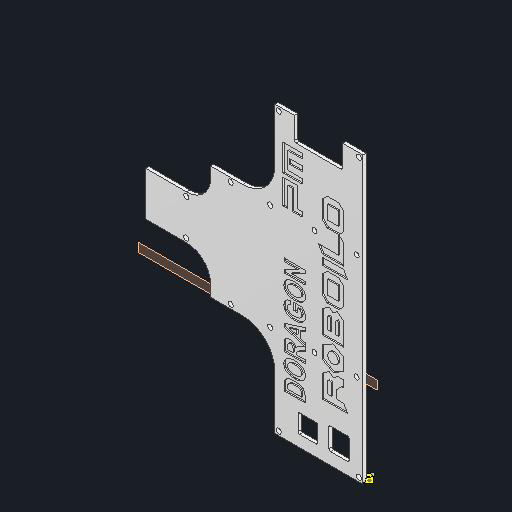
# Autodesk Inventor part: ceil
Saved by Autodesk Inventor 2023 (Build 270158000, 158)
## iProperties
Created: 2024-05-26
Part Number: ceil
Material: ABS Plastic
Document SubType Name: Modeling
Designer: szymo
Density: 1.06 g/cm^3
Appearance: Smooth - White
Mass: 26.6149 g
Surface Area: 293.171 cm^2
Volume: 25.1084 cm^3
TOTAL MASS: 0.0
Author: szymo
Autodesk Inventor part; units mm, degrees
ref_plane "YZ Plane" through (0, 0, 0) normal (1, 0, 0) x (0, 1, 0)
ref_plane "XZ Plane" through (0, 0, 0) normal (0, 1, 0) x (-1, 0, 0)
ref_plane "XY Plane" through (0, 0, 0) normal (0, 0, 1) x (1, 0, 0)
ref_plane "Work Plane1" through (-50.5, 0, 0) normal (0, 0, 1) x (1, 0, 0)
sketch "Sketch3" plane through (-50.5, 0, 0) normal (0, 0, 1) x (1, 0, 0)
  line L0 (135.5648, 0) -> (135.5648, 5.2284) projected
  line L1 (0, 5) -> (134.493, 5) projected
  line L2 (0, 0) -> (0, 5) projected
  line L3 (0, 71) -> (135.5648, 71) projected
  line L4 (0, 71) -> (0, 66) projected
  line L5 (0, 66) -> (135.5648, 66) projected
  line L6 (135.5648, 71) -> (135.5648, 66) projected
  line L7 (131.5648, 119.5) -> (134.5648, 119.5) projected
  line L8 (135.5648, 124.5) -> (135.5648, 120.5) projected
  line L9 (135.5648, 124.5) -> (51.5, 124.5) projected
  line L10 (86.5, 123.5) -> (129.5648, 123.5) projected
  line L11 (80.5, 122.5) -> (80.5, 120.5) projected
  line L12 (81.5, 119.5) -> (84.5, 119.5) projected
  line L13 (85.5, 122.5) -> (85.5, 120.5) projected
  line L14 (51.5, 123.5) -> (79.5, 123.5) projected
  line L15 (130.5648, 122.5) -> (130.5648, 120.5) projected
  line L16 (120.8148, 112) -> (120.8148, 123) projected
  line L17 (120.8148, 123) -> (94.8148, 123) projected
  line L18 (94.8148, 123) -> (94.8148, 112) projected
  line L19 (94.8148, 112) -> (120.8148, 112) projected
  line L20 (130.5648, -51.5) -> (130.5648, -49.5) projected
  line L21 (51.5, -52.5) -> (79.5, -52.5) projected
  line L22 (85.5, -51.5) -> (85.5, -49.5) projected
  line L23 (131.5648, -48.5) -> (134.5648, -48.5) projected
  line L24 (80.5, -51.5) -> (80.5, -49.5) projected
  line L25 (86.5, -52.5) -> (129.5648, -52.5) projected
  line L26 (135.5648, -53.5) -> (51.5, -53.5) projected
  line L27 (135.5648, -53.5) -> (135.5648, -49.5) projected
  line L28 (81.5, -48.5) -> (84.5, -48.5) projected
  line L29 (95.5648, -45.8) -> (95.5648, -35.2) projected
  line L30 (106.8648, -35.2) -> (95.5648, -35.2) projected
  line L31 (106.8648, -35.2) -> (106.8648, -45.8) projected
  line L32 (95.5648, -45.8) -> (106.8648, -45.8) projected
  circle A0 centre (90.4898, -49.075) radius 1.675 projected
  circle A1 centre (124.5398, -49.075) radius 1.675 projected
  line L33 (126.3648, -33.5) -> (126.3648, -45.5) projected
  line L34 (126.3648, -45.5) -> (114.7648, -45.5) projected
  line L35 (114.7648, -45.5) -> (114.7648, -33.5) projected
  line L36 (114.7648, -33.5) -> (86.8648, -33.5) projected
  line L37 (86.8648, -33.5) -> (86.8648, -52.5) projected
  line L38 (86.8648, -52.5) -> (128.0648, -52.5) projected
  line L39 (128.0648, -52.5) -> (128.0648, -33.5) projected
  line L40 (128.0648, -33.5) -> (126.3648, -33.5) projected
  line L41 (126.3648, -32.7) -> (114.7648, -32.7) projected
  line L42 (114.7648, -32.7) -> (114.7648, -45.5) projected
  line L43 (114.7648, -45.5) -> (126.3648, -45.5) projected
  line L44 (126.3648, -45.5) -> (126.3648, -32.7) projected
  line L45 (80.5, -53.5) -> (135.5648, -53.5)
  line L46 (135.5648, -53.5) -> (135.5648, 124.5)
  line L47 (135.5648, 124.5) -> (80.5, 124.5)
  line L48 (80.5, 124.5) -> (80.5, -53.5)
  line L49 (0, 22) -> (80.5, 22)
  line L50 (80.5, 22) -> (80.5, 49.5)
  line L51 (80.5, 49.5) -> (0, 49.5)
  line L52 (0, 49.5) -> (0, 22)
  line L53 (80.5, 22) -> (50.5, 22)
  line L54 (50.5, 22) -> (50.5, 0)
  line L55 (50.5, 0) -> (80.5, 0)
  line L56 (80.5, 0) -> (80.5, 22)
  line L57 (80.5, 46.5815) -> (80.5, 71)
  line L58 (80.5, 71) -> (50.5, 71)
  line L59 (50.5, 71) -> (50.5, 49.5)
  arc A2 (97.9124, 50.9) -> (98.0124, 51) centre (97.9124, 51) ccw projected
  line L60 (77.4124, 50.9) -> (97.9124, 50.9) projected
  arc A3 (77.3124, 51) -> (77.4124, 50.9) centre (77.4124, 51) ccw projected
  line L61 (77.3124, 65.5) -> (77.3124, 51) projected
  arc A4 (77.4124, 65.6) -> (77.3124, 65.5) centre (77.4124, 65.5) ccw projected
  line L62 (97.9124, 65.6) -> (77.4124, 65.6) projected
  arc A5 (98.0124, 65.5) -> (97.9124, 65.6) centre (97.9124, 65.5) ccw projected
  line L63 (98.0124, 51) -> (98.0124, 65.5) projected
  line L64 (96.2124, 63.7) -> (96.2124, 52.8) projected
  arc A6 (96.2124, 63.7) -> (95.9124, 64) centre (95.9124, 63.7) ccw projected
  line L65 (95.9124, 64) -> (95.8124, 64) projected
  line L66 (95.8124, 64) -> (95.3509, 64.55) projected
  line L67 (95.3509, 64.55) -> (94.9739, 64.55) projected
  line L68 (94.9739, 64.55) -> (94.5124, 64) projected
  line L69 (94.5124, 64) -> (90.8124, 64) projected
  line L70 (90.8124, 64) -> (90.8124, 64.35) projected
  line L71 (90.8124, 64.35) -> (89.5124, 64.35) projected
  line L72 (89.5124, 64) -> (89.5124, 64.35) projected
  line L73 (89.5124, 64) -> (85.8124, 64) projected
  line L74 (85.8124, 64) -> (85.8124, 64.35) projected
  line L75 (85.8124, 64.35) -> (84.5124, 64.35) projected
  line L76 (84.5124, 64) -> (84.5124, 64.35) projected
  line L77 (84.5124, 64) -> (80.8124, 64) projected
  line L78 (80.8124, 64) -> (80.3509, 64.55) projected
  line L79 (80.3509, 64.55) -> (79.9739, 64.55) projected
  line L80 (79.9739, 64.55) -> (79.5124, 64) projected
  line L81 (79.5124, 64) -> (79.4124, 64) projected
  arc A7 (79.4124, 64) -> (79.1124, 63.7) centre (79.4124, 63.7) ccw projected
  line L82 (79.1124, 63.7) -> (79.1124, 52.8) projected
  arc A8 (79.1124, 52.8) -> (79.4124, 52.5) centre (79.4124, 52.8) ccw projected
  line L83 (79.4124, 52.5) -> (79.5124, 52.5) projected
  line L84 (79.5124, 52.5) -> (79.9739, 51.95) projected
  line L85 (80.3509, 51.95) -> (79.9739, 51.95) projected
  line L86 (80.3509, 51.95) -> (80.8124, 52.5) projected
  line L87 (80.8124, 52.5) -> (84.5124, 52.5) projected
  line L88 (84.5124, 52.5) -> (84.5124, 52.15) projected
  line L89 (85.8124, 52.15) -> (84.5124, 52.15) projected
  line L90 (85.8124, 52.5) -> (85.8124, 52.15) projected
  line L91 (85.8124, 52.5) -> (89.5124, 52.5) projected
  line L92 (89.5124, 52.5) -> (89.5124, 52.15) projected
  line L93 (90.8124, 52.15) -> (89.5124, 52.15) projected
  line L94 (90.8124, 52.5) -> (90.8124, 52.15) projected
  line L95 (90.8124, 52.5) -> (94.5124, 52.5) projected
  line L96 (94.5124, 52.5) -> (94.9739, 51.95) projected
  line L97 (95.3509, 51.95) -> (94.9739, 51.95) projected
  line L98 (95.3509, 51.95) -> (95.8124, 52.5) projected
  line L99 (95.8124, 52.5) -> (95.9124, 52.5) projected
  arc A9 (95.9124, 52.5) -> (96.2124, 52.8) centre (95.9124, 52.8) ccw projected
  line L100 (78.1624, 55.35) -> (78.8624, 55.35) projected
  line L101 (78.8624, 55.35) -> (78.8624, 61.15) projected
  line L102 (78.1624, 61.15) -> (78.8624, 61.15) projected
  line L103 (78.1624, 61.15) -> (78.1624, 55.35) projected
  line L104 (97.1624, 61.15) -> (97.1624, 55.35) projected
  line L105 (96.4624, 61.15) -> (97.1624, 61.15) projected
  line L106 (96.4624, 55.35) -> (96.4624, 61.15) projected
  line L107 (96.4624, 55.35) -> (97.1624, 55.35) projected
  arc A10 (76.8124, 51) -> (77.4124, 50.4) centre (77.4124, 51) ccw
  line L108 (77.4124, 50.4) -> (97.9124, 50.4)
  arc A11 (97.9124, 50.4) -> (98.5124, 51) centre (97.9124, 51) ccw
  line L109 (98.5124, 51) -> (98.5124, 65.5)
  arc A12 (98.5124, 65.5) -> (97.9124, 66.1) centre (97.9124, 65.5) ccw
  line L110 (97.9124, 66.1) -> (77.4124, 66.1)
  arc A13 (77.4124, 66.1) -> (76.8124, 65.5) centre (77.4124, 65.5) ccw
  line L111 (76.8124, 65.5) -> (76.8124, 51)
  line L112 (95.0648, -34.7) -> (95.0648, -46.3)
  line L113 (95.0648, -46.3) -> (107.3648, -46.3)
  line L114 (107.3648, -46.3) -> (107.3648, -34.7)
  line L115 (107.3648, -34.7) -> (95.0648, -34.7)
  line L116 (114.2648, -45.5) -> (114.2648, -32.2)
  line L117 (114.2648, -32.2) -> (126.8648, -32.2)
  line L118 (126.8648, -32.2) -> (126.8648, -45.5)
  line L119 (126.3648, -46) -> (114.7648, -46)
  line L120 (92.8148, 110) -> (92.8148, 125)
  line L121 (92.8148, 125) -> (122.8148, 125)
  line L122 (122.8148, 125) -> (122.8148, 110)
  line L123 (122.8148, 110) -> (92.8148, 110)
  line L124 (114.2648, -45.5) -> (114.2648, -46)
  line L125 (114.2648, -46) -> (114.7648, -46)
  line L126 (126.3648, -46) -> (126.8648, -46)
  line L127 (126.8648, -46) -> (126.8648, -45.5)
  line L128 (51.5, -53.5) -> (51.5, -52.5) projected
  line L129 (51.5, 124.5) -> (51.5, 123.5) projected
  circle A14 centre (105.3205, 68.5) radius 1.75 projected
  circle A15 centre (53, 68.5) radius 1.75 projected
  circle A16 centre (77.648, 2.5) radius 1.75 projected
  circle A17 centre (131.5519, 2.5) radius 1.75 projected
  line L130 (50.5, 27) -> (0, 27) projected
  line L131 (0, 27) -> (0, 22) projected
  line L132 (50.5, 22) -> (0, 22) projected
  line L133 (50.5, 27) -> (50.5, 22) projected
  line L134 (50.5, 44.5) -> (0, 44.5) projected
  line L135 (50.5, 44.5) -> (50.5, 49.5) projected
  line L136 (50.5, 49.5) -> (0, 49.5) projected
  line L137 (0, 44.5) -> (0, 49.5) projected
  line L138 (50.5, 0) -> (40.5, 0)
  line L139 (40.5, 0) -> (40.5, 22)
  line L140 (40.5, 22) -> (50.5, 22)
  line L141 (50.5, 22) -> (50.5, 0)
  line L142 (50.5, 49.5) -> (40.5, 49.5)
  line L143 (40.5, 49.5) -> (40.5, 71)
  line L144 (40.5, 71) -> (50.5, 71)
  line L145 (50.5, 71) -> (50.5, 49.5)
  ellipse E0 centre (134.493, 7) end of major axis (136.8024, 7) minor radius 2 (134.493, 5) -> (135.5648, 5.2284) ccw projected
  circle A18 centre (25.25, 47) radius 1.75 projected
  circle A19 centre (25.25, 24.5) radius 1.75 projected
  line L146 (0, 0) -> (3.5, 0) projected
  line L147 (3.5, 0) -> (47, 0) projected
  line L148 (47, 0) -> (135.5648, 0) projected
  circle A20 centre (105.3205, 2.5) radius 1.75 projected
  circle A21 centre (53, 2.5) radius 1.75 projected
  arc A22 (81.5, -48.5) -> (80.5, -49.5) centre (81.5, -49.5) ccw projected
  arc A23 (79.5, -52.5) -> (80.5, -51.5) centre (79.5, -51.5) ccw projected
  arc A24 (135.5648, -49.5) -> (134.5648, -48.5) centre (134.5648, -49.5) ccw projected
  arc A25 (131.5648, -48.5) -> (130.5648, -49.5) centre (131.5648, -49.5) ccw projected
  arc A26 (129.5648, -52.5) -> (130.5648, -51.5) centre (129.5648, -51.5) ccw projected
  arc A27 (85.5, -51.5) -> (86.5, -52.5) centre (86.5, -51.5) ccw projected
  arc A28 (85.5, -49.5) -> (84.5, -48.5) centre (84.5, -49.5) ccw projected
  circle A29 centre (133.0648, -51) radius 1.75 projected
  circle A30 centre (83, -51) radius 1.75 projected
  arc A31 (86.5, 123.5) -> (85.5, 122.5) centre (86.5, 122.5) ccw projected
  arc A32 (130.5648, 122.5) -> (129.5648, 123.5) centre (129.5648, 122.5) ccw projected
  arc A33 (134.5648, 119.5) -> (135.5648, 120.5) centre (134.5648, 120.5) ccw projected
  arc A34 (80.5, 120.5) -> (81.5, 119.5) centre (81.5, 120.5) ccw projected
  arc A35 (84.5, 119.5) -> (85.5, 120.5) centre (84.5, 120.5) ccw projected
  arc A36 (130.5648, 120.5) -> (131.5648, 119.5) centre (131.5648, 120.5) ccw projected
  arc A37 (80.5, 122.5) -> (79.5, 123.5) centre (79.5, 122.5) ccw projected
  circle A38 centre (133.0648, 122) radius 1.75 projected
  circle A39 centre (83, 122) radius 1.75 projected
  point P0 (122.8148, 124.5)
  point P1 (92.8148, 124.5)
  point P2 (0, 44)
  point P3 (50.5, 44)
  point P4 (122.8148, 124.5)
  point P5 (122.8148, 123.5)
  point P6 (92.8148, 123.5)
  point P7 (92.8148, 124.5)
  point P8 (80.5, 123.5)
  point P9 (50.5, 66)
  point P10 (50.5, 5)
  point P11 (80.5, -52.5)
  point P12 (80.5, 66)
  point P13 (80.5, 5)
  point P14 (135.5648, 5)
  point P15 (80.5, 22)
  point P16 (50.5, 27)
  point P17 (0, 27)
  point P18 (80.5, -51.5)
  point P19 (77.0807, 66)
  point P20 (80.5, 66.1)
  point P21 (135.5648, 5.2284)
  point P22 (80.5, 50.4)
  point P23 (40.5, 5)
  point P24 (135.5648, 119.5)
  point P25 (80.5, 119.5)
  dimension "d16" = 0.5
  dimension "d17" = 0.5
  dimension "d18" = 0.5
  dimension "d19" = 0.5
  dimension "d20" = 2
  dimension "d191" = 10
  dimension "d192" = 10
  constraints: 86 end point, 12 parallel, 8 point on circle, 7 perpendicular, 7 point on line, 6 horizontal, 4 centre point, 2 collinear, 2 vertical, 17 other
  measures "d16" distance between parallel lines of L61 L111
  measures "d17" distance between parallel lines of L29 L112
  measures "d18" distance between parallel lines of L42 L116
  measures "d19" distance between parallel lines of L34 L119
  measures "d20" distance between parallel lines of L18 L120
  measures "d191" distance between parallel lines of L139 L54
  measures "d192" distance between parallel lines of L59 L143
extrude "Extrusion2" add sketch "Sketch3" along normal blind 2 contours L148 L48 L1 E0 L0 | L46 A24 L23 A25 L20 A26 L25 L39 L40 L118 L117 L116 L36 L37 A27 L22 A28 L28 A22 L48 L148 | E0 L1 L48 L108 A11 L109 A12 L5 L46 | L27 L26 L48 L24 A22 L28 A28 L22 A27 L25 A26 L20 A25 L23 A24 | L55 L54 L1 L48 | L5 A12 L110 L48 L3 L6 | L1 L54 L49 L48 | L138 L139 L1 L54 | A12 L109 A11 L108 L48 L60 A2 L63 A5 L62 L5 | L5 L48 L110 A12 | L3 L48 A34 L12 A35 L13 A31 L10 L120 L123 L122 A32 L15 A36 L7 A33 L46 | L1 L139 L49 L54 | L49 L133 L130 L52 L134 L135 L51 L48 | L48 L62 A4 L61 A3 L60 L108 A10 L111 A13 L5 | L5 A13 L110 L48 | L48 L110 A13 L5 L59 L3 | A33 L7 A36 L15 A32 L10 L122 L9 L8 | L49 L52 L130 L133 | A13 L111 A10 L108 L48 L51 L59 L5 | L62 A5 L63 A2 L60 L48 L86 L87 L88 L89 L90 L91 L92 L93 L94 L95 L96 L97 L98 L99 A9 L64 A6 L65 L66 L67 L68 L69 L70 L71 L72 L73 L74 L75 L76 L77 L78 | L48 L78 L79 L80 L81 A7 L82 A8 L83 L84 L85 L86 L60 A3 L61 A4 L62 | L59 L5 L143 L3 | L11 L48 L9 L120 L10 A31 L13 A35 L12 A34 | L59 L51 L143 L5 | L78 L77 L76 L75 L74 L73 L72 L71 L70 L69 L68 L67 L66 L65 A6 L64 A9 L99 L98 L97 L96 L95 L94 L93 L92 L91 L90 L89 L88 L87 L86 L48 | L48 L86 L85 L84 L83 A8 L82 A7 L81 L80 L79 L78 | L135 L134 L52 L51 | L25 L37 L36 L116 L124 L125 L119 L126 L127 L118 L40 L39 | A0 | A1 | L103 L102 L101 L100 | L104 L107 L106 L105 | A14 | A15 | A16 | A17 | A18 | A19 | A20 | A21 | A29 | A30 | A38 | A39
fillet "Fillet2" radius 1 10 edges at (44.5648, -46.3, 1) (44.5648, -34.7, 1) (56.8648, -34.7, 1) (56.8648, -46.3, 1) (63.7648, -46, 1) (63.7648, -32.2, 1) (76.3648, -32.2, 1) (76.3648, -46, 1) (42.3148, 110, 1) (72.3148, 110, 1)
fillet "Fillet3" radius 20 2 edges at (30, 71, 1) (30, 0, 1)
sketch "Sketch4" plane through (-50.5, 0, 2) normal (0, 0, 1) x (1, 0, 0)
  line L0 (130.5648, -51.5) -> (130.5648, -49.5) projected
  line L1 (51.5, -52.5) -> (79.5, -52.5) projected
  line L2 (85.5, -51.5) -> (85.5, -49.5) projected
  line L3 (131.5648, -48.5) -> (134.5648, -48.5) projected
  line L4 (80.5, -51.5) -> (80.5, -49.5) projected
  line L5 (86.5, -52.5) -> (129.5648, -52.5) projected
  line L6 (135.5648, -53.5) -> (51.5, -53.5) projected
  line L7 (135.5648, -53.5) -> (135.5648, -49.5) projected
  line L8 (81.5, -48.5) -> (84.5, -48.5) projected
  line L9 (131.5648, 119.5) -> (134.5648, 119.5) projected
  line L10 (135.5648, 124.5) -> (135.5648, 120.5) projected
  line L11 (135.5648, 124.5) -> (51.5, 124.5) projected
  line L12 (86.5, 123.5) -> (129.5648, 123.5) projected
  line L13 (80.5, 122.5) -> (80.5, 120.5) projected
  line L14 (81.5, 119.5) -> (84.5, 119.5) projected
  line L15 (85.5, 122.5) -> (85.5, 120.5) projected
  line L16 (51.5, 123.5) -> (79.5, 123.5) projected
  line L17 (130.5648, 122.5) -> (130.5648, 120.5) projected
  line L18 (51.5, 124.5) -> (51.5, 123.5) projected
  line L19 (51.5, -53.5) -> (51.5, -52.5) projected
  line L20 (50.5, 27) -> (0, 27) projected
  line L21 (0, 27) -> (0, 22) projected
  line L22 (50.5, 22) -> (0, 22) projected
  line L23 (50.5, 27) -> (50.5, 22) projected
  line L24 (50.5, 44.5) -> (0, 44.5) projected
  line L25 (50.5, 44.5) -> (50.5, 49.5) projected
  line L26 (50.5, 49.5) -> (0, 49.5) projected
  line L27 (0, 44.5) -> (0, 49.5) projected
  circle A0 centre (77.648, 68.5) radius 1.75 projected
  circle A1 centre (105.3205, 68.5) radius 1.75 projected
  circle A2 centre (53, 68.5) radius 1.75 projected
  circle A3 centre (131.5519, 68.5) radius 1.75 projected
  line L28 (0, 71) -> (0, 66) projected
  line L29 (0, 66) -> (134.493, 66) projected
  line L30 (135.5648, 71) -> (135.5648, 65.7716) projected
  circle A4 centre (77.648, 2.5) radius 1.75 projected
  circle A5 centre (105.3205, 2.5) radius 1.75 projected
  circle A6 centre (53, 2.5) radius 1.75 projected
  circle A7 centre (131.5519, 2.5) radius 1.75 projected
  line L31 (135.5648, 0) -> (135.5648, 5.2284) projected
  line L32 (0, 5) -> (134.493, 5) projected
  line L33 (0, 0) -> (0, 5) projected
  ellipse E0 centre (134.493, 64) end of major axis (136.8024, 64) minor radius 2 (135.5648, 65.7716) -> (134.493, 66) ccw projected
  ellipse E1 centre (134.493, 7) end of major axis (136.8024, 7) minor radius 2 (134.493, 5) -> (135.5648, 5.2284) ccw projected
  circle A8 centre (25.25, 47) radius 1.75 projected
  circle A9 centre (25.25, 24.5) radius 1.75 projected
  line L34 (0, 71) -> (3.5, 71) projected
  line L35 (47, 71) -> (135.5648, 71) projected
  line L36 (3.5, 71) -> (47, 71) projected
  line L37 (0, 0) -> (3.5, 0) projected
  line L38 (3.5, 0) -> (47, 0) projected
  line L39 (47, 0) -> (135.5648, 0) projected
  arc A10 (86.5, 123.5) -> (85.5, 122.5) centre (86.5, 122.5) ccw projected
  arc A11 (130.5648, 122.5) -> (129.5648, 123.5) centre (129.5648, 122.5) ccw projected
  arc A12 (134.5648, 119.5) -> (135.5648, 120.5) centre (134.5648, 120.5) ccw projected
  arc A13 (81.5, -48.5) -> (80.5, -49.5) centre (81.5, -49.5) ccw projected
  arc A14 (79.5, -52.5) -> (80.5, -51.5) centre (79.5, -51.5) ccw projected
  arc A15 (135.5648, -49.5) -> (134.5648, -48.5) centre (134.5648, -49.5) ccw projected
  arc A16 (131.5648, -48.5) -> (130.5648, -49.5) centre (131.5648, -49.5) ccw projected
  arc A17 (129.5648, -52.5) -> (130.5648, -51.5) centre (129.5648, -51.5) ccw projected
  arc A18 (85.5, -51.5) -> (86.5, -52.5) centre (86.5, -51.5) ccw projected
  arc A19 (85.5, -49.5) -> (84.5, -48.5) centre (84.5, -49.5) ccw projected
  circle A20 centre (133.0648, -51) radius 1.75 projected
  circle A21 centre (83, -51) radius 1.75 projected
  arc A22 (80.5, 120.5) -> (81.5, 119.5) centre (81.5, 120.5) ccw projected
  arc A23 (84.5, 119.5) -> (85.5, 120.5) centre (84.5, 120.5) ccw projected
  arc A24 (130.5648, 120.5) -> (131.5648, 119.5) centre (131.5648, 120.5) ccw projected
  arc A25 (80.5, 122.5) -> (79.5, 123.5) centre (79.5, 122.5) ccw projected
  circle A26 centre (133.0648, 122) radius 1.75 projected
  circle A27 centre (83, 122) radius 1.75 projected
  point P0 (50.5, 0)
  point P1 (83, -51)
  point P2 (133.0648, -51)
  point P3 (0, 44)
  point P4 (50.5, 44)
  point P5 (50.5, 27)
  point P6 (0, 27)
  constraints: 10 coincident, 2 other
hole "Hole2" at (32.5, -51, 2) at (82.5648, -51, 2) at (82.5648, 122, 2) at (32.5, 122, 2) at (54.8205, 68.5, 2) at (2.5, 2.5, 2) at (2.5, 68.5, 2) at (54.8205, 2.5, 2) at (81.0519, 2.5, 2) at (81.0519, 68.5, 2) at (27.148, 68.5, 2) at (27.148, 2.5, 2) at (-25.25, 24.5, 2) at (-25.25, 47, 2) direction (0, 0, -1) diameter 3.2 end through all clearance for "Countersunk Flat Head Screw ISO 2009/7046" size "M2.5" standard "ISO"
fillet "Fillet4" radius 15 2 edges at (-10, 22, 1) (-10, 49.5, 1)
sketch "Sketch5" plane through (-50.5, 0, 2) normal (0, 0, 1) x (1, 0, 0)
  line L0 (80.5, -53.5) -> (135.5648, -53.5) projected
  line L1 (135.5648, -53.5) -> (135.5648, 124.5) projected
  line L2 (60.5, 71) -> (40.5, 71) projected
  line L3 (25.5, 49.5) -> (0, 49.5) projected
  line L4 (0, 49.5) -> (0, 22) projected
  line L5 (0, 22) -> (25.5, 22) projected
  line L6 (105.3205, -31.7) -> (105.3205, 48.4) construction
  line L7 (105.3205, 48.4) -> (80.5, 48.4) construction
  line L8 (80.5, 48.4) -> (80.5, -31.7) construction
  line L9 (80.5, -31.7) -> (105.3205, -31.7) construction
  line L10 (110.1651, 28.6458) -> (110.1651, 14.5717) projected
  line L11 (119.2148, -10.52) -> (122.2141, -7.4431) projected
  line L12 (122.2141, -7.4431) -> (123.5648, -7.4431) projected
  line L13 (123.5648, -7.4431) -> (123.5648, -3.1151) projected
  line L14 (123.5648, -3.1151) -> (119.5551, -3.1151) projected
  line L15 (119.5551, -3.1151) -> (117.3584, -5.3021) projected
  line L16 (117.3584, -5.3021) -> (114.3535, -3.0659) projected
  line L17 (114.3535, -3.0659) -> (110.1651, -6.1782) projected
  line L18 (110.1651, -6.1782) -> (110.1651, -20.0711) projected
  line L19 (110.1651, -20.0711) -> (125.9602, -20.0711) projected
  line L20 (125.9602, -20.0711) -> (123.4807, -15.7431) projected
  line L21 (123.4807, -15.7431) -> (119.2148, -15.7431) projected
  line L22 (119.2148, -15.7431) -> (119.2148, -10.52) projected
  line L23 (114.6271, -7.6036) -> (115.8612, -8.5098) projected
  line L24 (115.8612, -8.5098) -> (115.8612, -15.7431) projected
  line L25 (115.8612, -15.7431) -> (113.4584, -15.7431) projected
  line L26 (113.4584, -15.7431) -> (113.4584, -8.4973) projected
  line L27 (113.4584, -8.4973) -> (114.6271, -7.6036) projected
  line L28 (123.5648, 1.4254) -> (123.5648, 9.1617) projected
  line L29 (123.5648, 9.1617) -> (116.8649, 13.0299) projected
  line L30 (116.8649, 13.0299) -> (110.1651, 9.1617) projected
  line L31 (110.1651, 9.1617) -> (110.1651, 1.4254) projected
  line L32 (110.1651, 1.4254) -> (116.8649, -2.4427) projected
  line L33 (116.8649, -2.4427) -> (123.5648, 1.4254) projected
  circle A0 centre (116.8649, 5.2936) radius 3.3 projected
  line L34 (123.5848, 14.5717) -> (123.5848, 28.6458) projected
  line L35 (123.5848, 28.6458) -> (119.3867, 31.747) projected
  line L36 (119.3867, 31.747) -> (116.875, 29.8983) projected
  line L37 (116.875, 29.8983) -> (114.3632, 31.747) projected
  line L38 (114.3632, 31.747) -> (110.1651, 28.6458) projected
  line L39 (110.1651, 28.6458) -> (110.1651, 14.5717) projected
  line L40 (110.1651, 14.5717) -> (123.5848, 14.5717) projected
  line L41 (115.3489, 26.1486) -> (115.3489, 18.8997) projected
  line L42 (115.3489, 18.8997) -> (113.4785, 18.8997) projected
  line L43 (113.4785, 18.8997) -> (113.4785, 26.1539) projected
  line L44 (113.4785, 26.1539) -> (114.3691, 26.9374) projected
  line L45 (114.3691, 26.9374) -> (115.3489, 26.1486) projected
  line L46 (118.4011, 18.8997) -> (118.4011, 26.1486) projected
  line L47 (118.4011, 26.1486) -> (119.3808, 26.9374) projected
  line L48 (119.3808, 26.9374) -> (120.2715, 26.1539) projected
  line L49 (120.2715, 26.1539) -> (120.2715, 18.8997) projected
  line L50 (120.2715, 18.8997) -> (118.4011, 18.8997) projected
  line L51 (120.494, 33.3579) -> (123.5648, 36.4286) projected
  line L52 (123.5648, 36.4286) -> (123.5648, 47.4441) projected
  line L53 (123.5648, 47.4441) -> (120.494, 50.5148) projected
  line L54 (120.494, 50.5148) -> (113.2358, 50.5148) projected
  line L55 (113.2358, 50.5148) -> (110.1651, 47.4441) projected
  line L56 (110.1651, 47.4441) -> (110.1651, 36.4286) projected
  line L57 (110.1651, 36.4286) -> (113.2358, 33.3579) projected
  line L58 (113.2358, 33.3579) -> (120.494, 33.3579) projected
  line L59 (120.2715, 37.686) -> (113.4584, 37.686) projected
  line L60 (113.4584, 37.686) -> (113.4584, 46.1868) projected
  line L61 (113.4584, 46.1868) -> (120.2715, 46.1868) projected
  line L62 (120.2715, 46.1868) -> (120.2715, 37.686) projected
  line L63 (125.9586, 52.2145) -> (123.5013, 56.5425) projected
  line L64 (123.5013, 56.5425) -> (110.1651, 56.5425) projected
  line L65 (110.1651, 56.5425) -> (110.1651, 52.2145) projected
  line L66 (110.1651, 52.2145) -> (125.9586, 52.2145) projected
  line L67 (123.5648, 88.0003) -> (120.494, 91.071) projected
  line L68 (120.494, 91.071) -> (113.2358, 91.071) projected
  line L69 (113.2358, 91.071) -> (110.1651, 88.0003) projected
  line L70 (110.1651, 88.0003) -> (110.1651, 76.9848) projected
  line L71 (110.1651, 76.9848) -> (113.2358, 73.9141) projected
  line L72 (113.2358, 73.9141) -> (120.2715, 73.9141) projected
  line L73 (120.2715, 73.9141) -> (120.2715, 62.7008) projected
  line L74 (120.2715, 62.7008) -> (107.738, 62.7008) projected
  line L75 (107.738, 62.7008) -> (110.2396, 58.3727) projected
  line L76 (110.2396, 58.3727) -> (123.5848, 58.3727) projected
  line L77 (123.5848, 58.3727) -> (123.5848, 70.8415) projected
  line L78 (123.5848, 70.8415) -> (120.5032, 73.9232) projected
  line L79 (120.5032, 73.9232) -> (123.5648, 76.9848) projected
  line L80 (123.5648, 76.9848) -> (123.5648, 88.0003) projected
  line L81 (120.2715, 78.2421) -> (113.4584, 78.2421) projected
  line L82 (113.4584, 78.2421) -> (113.4584, 86.743) projected
  line L83 (113.4584, 86.743) -> (120.2715, 86.743) projected
  line L84 (120.2715, 86.743) -> (120.2715, 78.2421) projected
  line L85 (91.5024, 71.975) -> (97.5262, 71.975) projected
  line L86 (97.5262, 71.975) -> (97.5262, 74.9242) projected
  line L87 (97.5262, 74.9242) -> (94.45, 74.9242) projected
  line L88 (94.45, 74.9242) -> (94.45, 87.525) projected
  line L89 (94.45, 87.525) -> (85.5, 87.525) projected
  line L90 (85.5, 87.525) -> (85.5, 71.975) projected
  line L91 (85.5, 71.975) -> (88.675, 71.975) projected
  line L92 (88.675, 71.975) -> (88.675, 84.4887) projected
  line L93 (88.675, 84.4887) -> (91.5024, 84.4887) projected
  line L94 (91.5024, 84.4887) -> (91.5024, 71.975) projected
  line L95 (85.5, 106.5) -> (85.5, 89.825) projected
  line L96 (85.5, 89.825) -> (97.6, 89.825) projected
  line L97 (97.6, 89.825) -> (97.6, 92.775) projected
  line L98 (97.6, 92.775) -> (88.6, 92.775) projected
  line L99 (88.6, 92.775) -> (88.6, 103.4705) projected
  line L100 (88.6, 103.4705) -> (97.5254, 103.4705) projected
  line L101 (97.5254, 103.4705) -> (97.5254, 106.5) projected
  line L102 (97.5254, 106.5) -> (85.5, 106.5) projected
  line L103 (89.7, 99.675) -> (89.7, 96.575) projected
  line L104 (89.7, 96.575) -> (97.6, 96.575) projected
  line L105 (97.6, 96.575) -> (97.6, 99.675) projected
  line L106 (97.6, 99.675) -> (89.7, 99.675) projected
  line L107 (80.5, -20) -> (80.5, -53.5) projected
  line L108 (80.5, 124.5) -> (80.5, 91) projected
  arc A1 (60.5, 71) -> (80.5, 91) centre (60.5, 91) ccw projected
  circle A2 centre (105.3205, 2.5) radius 1.6 projected
  line L109 (40.5, 71) -> (40.5, 64.5) projected
  line L110 (40.5, 7) -> (40.5, 0) projected
  arc A3 (25.5, 49.5) -> (40.5, 64.5) centre (25.5, 64.5) ccw projected
  arc A4 (40.5, 7) -> (25.5, 22) centre (25.5, 7) ccw projected
  line L111 (40.5, 0) -> (60.5, 0) projected
  arc A5 (80.5, -20) -> (60.5, 0) centre (60.5, -20) ccw projected
  line L112 (135.5648, 124.5) -> (122.8148, 124.5) projected
  line L113 (122.8148, 124.5) -> (122.8148, 111) projected
  arc A6 (121.8148, 110) -> (122.8148, 111) centre (121.8148, 111) ccw projected
  line L114 (121.8148, 110) -> (93.8148, 110) projected
  arc A7 (92.8148, 111) -> (93.8148, 110) centre (93.8148, 111) ccw projected
  line L115 (92.8148, 111) -> (92.8148, 124.5) projected
  line L116 (92.8148, 124.5) -> (80.5, 124.5) projected
  line L117 (86.4102, -27.5982) -> (86.4102, -23.8627)
  spline S0 degree 2 poles (86.4102, -23.8627) (86.4102, -22.5944) (86.6579, -21.9305) knots 0 0 0 1 1 1
  spline S1 degree 2 poles (86.6579, -21.9305) (86.9948, -21.0387) (88.7189, -19.7704) (91.206, -19.1066) (93.039, -19.1066) knots 0 0 0 1 2 3 3 3
  spline S2 degree 2 poles (93.039, -19.1066) (94.6442, -19.1066) (95.8035, -19.4137) knots 0 0 0 1 1 1
  spline S3 degree 2 poles (95.8035, -19.4137) (97.2204, -19.8002) (98.1023, -20.5037) knots 0 0 0 1 1 1
  spline S4 degree 2 poles (98.1023, -20.5037) (98.7662, -21.0387) (99.1328, -21.9404) knots 0 0 0 1 1 1
  spline S5 degree 2 poles (99.1328, -21.9404) (99.4102, -22.6142) (99.4102, -23.7537) knots 0 0 0 1 1 1
  line L118 (99.4102, -23.7537) -> (99.4102, -27.5982)
  line L119 (99.4102, -27.5982) -> (86.4102, -27.5982)
  line L120 (88.6099, -25.5471) -> (97.2105, -25.5471)
  line L121 (97.2105, -25.5471) -> (97.2105, -24.0212)
  spline S6 degree 2 poles (97.2105, -24.0212) (97.2105, -23.1691) (97.0817, -22.7826) knots 0 0 0 1 1 1
  spline S7 degree 2 poles (97.0817, -22.7826) (96.9232, -22.2872) (96.1701, -21.6332) (94.4163, -21.2171) (92.9102, -21.2171) knots 0 0 0 1 2 3 3 3
  spline S8 degree 2 poles (92.9102, -21.2171) (91.4041, -21.2171) (89.799, -21.6332) (88.8973, -22.3764) (88.7387, -22.9511) knots 0 0 0 1 2 3 3 3
  spline S9 degree 2 poles (88.7387, -22.9511) (88.6099, -23.3771) (88.6099, -24.6256) knots 0 0 0 1 1 1
  line L122 (88.6099, -24.6256) -> (88.6099, -25.5471)
  spline S10 degree 2 poles (92.9895, -17.7887) (91.0078, -17.7887) (89.6602, -17.323) knots 0 0 0 1 1 1
  spline S11 degree 2 poles (89.6602, -17.323) (88.6694, -16.9762) (87.084, -15.7773) (86.7075, -15.0738) knots 0 0 0 1 2 2 2
  spline S12 degree 2 poles (86.7075, -15.0738) (86.1922, -14.1226) (86.1922, -12.884) knots 0 0 0 1 1 1
  spline S13 degree 2 poles (86.1922, -12.884) (86.1922, -10.6447) (89.7593, -7.9495) (92.9301, -7.9495) knots 0 0 0 1 2 2 2
  spline S14 degree 2 poles (92.9301, -7.9495) (96.0711, -7.9495) (99.6282, -10.6248) (99.6282, -12.8543) knots 0 0 0 1 2 2 2
  spline S15 degree 2 poles (99.6282, -12.8543) (99.6282, -15.1134) (96.0909, -17.7887) (92.9895, -17.7887) knots 0 0 0 1 2 2 2
  spline S16 degree 2 poles (92.9003, -15.6782) (95.1099, -15.6782) (97.3889, -14.0829) (97.3889, -12.8543) knots 0 0 0 1 2 2 2
  spline S17 degree 2 poles (97.3889, -12.8543) (97.3889, -11.6355) (95.1297, -10.0601) (92.8706, -10.0601) knots 0 0 0 1 2 2 2
  spline S18 degree 2 poles (92.8706, -10.0601) (90.6313, -10.0601) (88.4316, -11.5959) (88.4316, -12.8543) knots 0 0 0 1 2 2 2
  spline S19 degree 2 poles (88.4316, -12.8543) (88.4316, -14.1226) (90.661, -15.6782) (92.9003, -15.6782) knots 0 0 0 1 2 2 2
  line L123 (99.4102, -6.3543) -> (86.4102, -6.3543)
  line L124 (86.4102, -6.3543) -> (86.4102, -2.0441)
  spline S20 degree 2 poles (86.4102, -2.0441) (86.4102, -0.4191) (87.1137, 1.0573) (88.8973, 1.9392) (90.0566, 1.9392) knots 0 0 0 1 2 3 3 3
  spline S21 degree 2 poles (90.0566, 1.9392) (91.5131, 1.9392) (93.4255, 0.6015) (93.6732, -0.7361) knots 0 0 0 1 2 2 2
  spline S22 degree 2 poles (93.6732, -0.7361) (94.1686, -0.0723) (95.3576, 0.7898) (96.8736, 1.523) knots 0 0 0 1 2 2 2
  line L125 (96.8736, 1.523) -> (99.4102, 2.7616)
  line L126 (99.4102, 2.7616) -> (99.4102, 0.3142)
  line L127 (99.4102, 0.3142) -> (96.5764, -1.1622)
  spline S23 degree 2 poles (96.5764, -1.1622) (95.0604, -1.9549) (94.2776, -2.5296) (93.9804, -3.1835) (93.9804, -3.887) knots 0 0 0 1 2 3 3 3
  line L128 (93.9804, -3.887) -> (93.9804, -4.3032)
  line L129 (93.9804, -4.3032) -> (99.4102, -4.3032)
  line L130 (99.4102, -4.3032) -> (99.4102, -6.3543)
  line L131 (91.9095, -4.3032) -> (91.9095, -2.7872)
  spline S24 degree 2 poles (91.9095, -2.7872) (91.9095, -1.3207) (91.5924, -0.5875) (90.8096, -0.1713) (90.225, -0.1713) knots 0 0 0 1 2 3 3 3
  spline S25 degree 2 poles (90.225, -0.1713) (89.5711, -0.1713) (88.7586, -0.7163) (88.6496, -1.2117) knots 0 0 0 1 2 2 2
  spline S26 degree 2 poles (88.6496, -1.2117) (88.6099, -1.4595) (88.6099, -2.7079) knots 0 0 0 1 1 1
  line L132 (88.6099, -2.7079) -> (88.6099, -4.3032)
  line L133 (88.6099, -4.3032) -> (91.9095, -4.3032)
  line L134 (99.4102, 13.0169) -> (99.4102, 10.7875)
  line L135 (99.4102, 10.7875) -> (96.4575, 9.9056)
  line L136 (96.4575, 9.9056) -> (96.4575, 5.853)
  line L137 (96.4575, 5.853) -> (99.4102, 5.0108)
  line L138 (99.4102, 5.0108) -> (99.4102, 2.8409)
  line L139 (99.4102, 2.8409) -> (86.4102, 6.7845)
  line L140 (86.4102, 6.7845) -> (86.4102, 8.9643)
  line L141 (86.4102, 8.9643) -> (99.4102, 13.0169)
  line L142 (94.2578, 9.2517) -> (89.4422, 7.8546)
  line L143 (89.4422, 7.8546) -> (94.2578, 6.4773)
  line L144 (94.2578, 6.4773) -> (94.2578, 9.2517)
  line L145 (94.6442, 18.8134) -> (92.4445, 18.8134)
  line L146 (92.4445, 18.8134) -> (92.4445, 23.2227)
  line L147 (92.4445, 23.2227) -> (97.6168, 23.2227)
  spline S27 degree 2 poles (97.6168, 23.2227) (98.4194, 22.5787) (99.6282, 20.1412) (99.6282, 18.8828) knots 0 0 0 1 2 2 2
  spline S28 degree 2 poles (99.6282, 18.8828) (99.6282, 17.2974) (97.914, 14.9293) (94.7334, 13.7402) (92.8706, 13.7402) knots 0 0 0 1 2 3 3 3
  spline S29 degree 2 poles (92.8706, 13.7402) (90.8394, 13.7402) (87.6785, 15.068) (86.8363, 16.3462) knots 0 0 0 1 2 2 2
  spline S30 degree 2 poles (86.8363, 16.3462) (86.1922, 17.3271) (86.1922, 18.7738) knots 0 0 0 1 1 1
  spline S31 degree 2 poles (86.1922, 18.7738) (86.1922, 20.6663) (88.2235, 22.7867) (90.0169, 23.0939) knots 0 0 0 1 2 2 2
  line L148 (90.0169, 23.0939) -> (90.5025, 21.0627)
  spline S32 degree 2 poles (90.5025, 21.0627) (89.5413, 20.8447) (88.4316, 19.6655) (88.4316, 18.7738) knots 0 0 0 1 2 2 2
  spline S33 degree 2 poles (88.4316, 18.7738) (88.4316, 17.4361) (90.6115, 15.8508) (92.7616, 15.8508) knots 0 0 0 1 2 2 2
  spline S34 degree 2 poles (92.7616, 15.8508) (95.0703, 15.8508) (97.3889, 17.4559) (97.3889, 18.754) knots 0 0 0 1 2 2 2
  spline S35 degree 2 poles (97.3889, 18.754) (97.3889, 19.398) (96.7448, 20.6861) (96.289, 21.1518) knots 0 0 0 1 2 2 2
  line L149 (96.289, 21.1518) -> (94.6442, 21.1518)
  line L150 (94.6442, 21.1518) -> (94.6442, 18.8134)
  spline S36 degree 2 poles (92.9895, 24.6991) (91.0078, 24.6991) (89.6602, 25.1648) knots 0 0 0 1 1 1
  spline S37 degree 2 poles (89.6602, 25.1648) (88.6694, 25.5116) (87.084, 26.7105) (86.7075, 27.414) knots 0 0 0 1 2 2 2
  spline S38 degree 2 poles (86.7075, 27.414) (86.1922, 28.3652) (86.1922, 29.6038) knots 0 0 0 1 1 1
  spline S39 degree 2 poles (86.1922, 29.6038) (86.1922, 31.8431) (89.7593, 34.5383) (92.9301, 34.5383) knots 0 0 0 1 2 2 2
  spline S40 degree 2 poles (92.9301, 34.5383) (96.0711, 34.5383) (99.6282, 31.863) (99.6282, 29.6335) knots 0 0 0 1 2 2 2
  spline S41 degree 2 poles (99.6282, 29.6335) (99.6282, 27.3744) (96.0909, 24.6991) (92.9895, 24.6991) knots 0 0 0 1 2 2 2
  spline S42 degree 2 poles (92.9003, 26.8096) (95.1099, 26.8096) (97.3889, 28.4049) (97.3889, 29.6335) knots 0 0 0 1 2 2 2
  spline S43 degree 2 poles (97.3889, 29.6335) (97.3889, 30.8523) (95.1297, 32.4277) (92.8706, 32.4277) knots 0 0 0 1 2 2 2
  spline S44 degree 2 poles (92.8706, 32.4277) (90.6313, 32.4277) (88.4316, 30.8919) (88.4316, 29.6335) knots 0 0 0 1 2 2 2
  spline S45 degree 2 poles (88.4316, 29.6335) (88.4316, 28.3652) (90.661, 26.8096) (92.9003, 26.8096) knots 0 0 0 1 2 2 2
  line L151 (99.4102, 36.1534) -> (86.4102, 36.1534)
  line L152 (86.4102, 36.1534) -> (86.4102, 38.1351)
  line L153 (86.4102, 38.1351) -> (95.1297, 42.3066)
  line L154 (95.1297, 42.3066) -> (86.4102, 42.3066)
  line L155 (86.4102, 42.3066) -> (86.4102, 44.1991)
  line L156 (86.4102, 44.1991) -> (99.4102, 44.1991)
  line L157 (99.4102, 44.1991) -> (99.4102, 42.1579)
  line L158 (99.4102, 42.1579) -> (90.8889, 38.0459)
  line L159 (90.8889, 38.0459) -> (99.4102, 38.0459)
  line L160 (99.4102, 38.0459) -> (99.4102, 36.1534)
  point P0 (50.5, 0)
  point P1 (80.5, -20)
  constraints: 2 point on line, 2 other
extrude "Extrusion4" cut sketch "Sketch5" against normal blind 0.8 contours L38 L37 L36 L35 L34 L40 L10 | L22 L21 L20 L19 L18 L17 L16 L15 L14 L13 L12 L11 | L33 L32 L31 L30 L29 L28 | L58 L57 L56 L55 L54 L53 L52 L51 | L66 L65 L64 L63 | L80 L79 L78 L77 L76 L75 L74 L73 L72 L71 L70 L69 L68 L67 | L94 L93 L92 L91 L90 L89 L88 L87 L86 L85 | L102 L101 L100 L99 L98 L97 L96 L95 | L106 L105 L104 L103 | L117 S0 S1 S2 S3 S4 S5 L118 L119 | S10 S11 S12 S13 S14 S15 | L123 L124 S20 S21 S22 L125 L126 L127 S23 L128 L129 L130 | L134 L135 L136 L137 L138 L139 L140 L141 | L145 L146 L147 S27 S28 S29 S30 S31 L148 S32 S33 S34 S35 L149 L150 | S36 S37 S38 S39 S40 S41 | L151 L152 L153 L154 L155 L156 L157 L158 L159 L160
body "Solid2"
